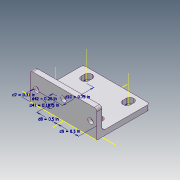
# Autodesk Inventor part: J005358
Saved by Autodesk Inventor 2015 SP1 (Build 190203100, 203)
## iProperties
Created: 2015-08-10
Material: ALUMINUM, 6061-T651
Vendor: HHMI: JRC - ID&F
Document SubType Name: Modeling
Designer: ARNOLDJ
Density: 2.7 g/cm^3
Appearance: Metal-AL-6061 (Machined)
Mass: 8.98458 g
Surface Area: 27.6253 cm^2
Volume: 3.32762 cm^3
Description: MOUNT FOR STEEL PART ON ROTARY LOCK
Project: P-201804
Part Number: J005358
RuleStatus: InUse
AfterDocSave0: file://Part Number Cleaner
LAB/DEPT: SVOBODA (LAB)
REQUESTING SCIENTIST: SOFRONIEW, NICK
SURFACE ROUGHNESS: 63 Ra
DESIGN DEPARTMENT: HHMI: JRC - ID&F
SPECIAL FINISH: NONE
ALTERED ITEM PART NUMBER: N/A
ALTERED ITEM VENDOR: N/A
ALTERED ITEM DESCRIPTION: N/A
Revision Number: -
Autodesk Inventor part; units mm, degrees
ref_plane "YZ Plane" through (0, 0, 0) normal (1, 0, 0) x (0, 1, 0)
ref_plane "XY Plane" through (0, 0, 0) normal (0, 0, 1) x (1, 0, 0)
sketch "Sketch1" plane through (0, 0, 0) normal (0, 0, 1) x (1, 0, 0)
  line L0 (20.32, -8.255) -> (-20.32, -8.255)
  line L1 (-20.32, -8.255) -> (-20.32, 8.255)
  line L2 (-20.32, 8.255) -> (20.32, 8.255)
  line L3 (20.32, 8.255) -> (20.32, -8.255)
  line L4 (20.32, -8.255) -> (-20.32, 8.255) construction
  line L5 (-20.32, -8.255) -> (20.32, 8.255) construction
  point P0 (0, 0)
  dimension "d0" = 40.64
  dimension "d1" = 16.51
  constraints: 12 end point, 2 midpoint, 2 parallel, 1 horizontal, 1 perpendicular
  measures "d0" distance of L1.end L2.end
  measures "d1" distance of L0.end L1.end
extrude "Extrusion1" add sketch "Sketch1" along normal blind 3.175
sketch "Sketch2" plane through (0, 0, 0) normal (0, 0, 1) x (1, 0, 0)
  line L0 (20.32, 8.255) -> (20.32, -8.255) projected
  line L1 (-20.32, -8.255) -> (-20.32, 8.255) projected
  line L2 (20.32, -8.255) -> (-20.32, -8.255) projected
  line L3 (20.32, -8.255) -> (-20.32, -8.255)
  line L4 (-20.32, -8.255) -> (-20.32, -5.08)
  line L5 (-20.32, -5.08) -> (20.32, -5.08)
  line L6 (20.32, -5.08) -> (20.32, -8.255)
  point P0 (0, 0)
  dimension "d4" = 3.175
  constraints: 8 end point, 2 parallel, 1 horizontal, 1 perpendicular, 1 point on line
  measures "d4" distance between parallel lines of L2 L5
extrude "Extrusion2" add sketch "Sketch2" against normal blind 29.21
sketch "Sketch3" plane through (-20.32, -8.255, 3.175) normal (0, -1, 0) x (1, 0, 0)
  line L0 (20.32, 6.477) -> (20.32, -38.862) projected
  line L1 (-8.128, -3.175) -> (48.768, -3.175) projected
  line L2 (0, 0) -> (40.64, 0) projected
  line L3 (10.0012, -11.176) -> (5.2387, -11.176)
  line L4 (5.2387, -11.176) -> (5.2387, -4.572)
  line L5 (5.2387, -4.572) -> (10.0012, -4.572)
  line L6 (10.0012, -4.572) -> (10.0012, -11.176)
  line L7 (10.0012, -11.176) -> (5.2387, -4.572) construction
  line L8 (5.2387, -11.176) -> (10.0012, -4.572) construction
  line L9 (35.4012, -11.176) -> (30.6387, -11.176)
  line L10 (30.6387, -11.176) -> (30.6387, -4.572)
  line L11 (30.6387, -4.572) -> (35.4012, -4.572)
  line L12 (35.4012, -4.572) -> (35.4012, -11.176)
  line L13 (35.4012, -11.176) -> (30.6387, -4.572) construction
  line L14 (30.6387, -11.176) -> (35.4012, -4.572) construction
  line L15 (35.4012, -30.226) -> (30.6387, -30.226)
  line L16 (30.6387, -30.226) -> (30.6387, -23.622)
  line L17 (30.6387, -23.622) -> (35.4012, -23.622)
  line L18 (35.4012, -23.622) -> (35.4012, -30.226)
  line L19 (35.4012, -30.226) -> (30.6387, -23.622) construction
  line L20 (30.6387, -30.226) -> (35.4012, -23.622) construction
  line L21 (5.2387, -30.226) -> (10.0012, -30.226)
  line L22 (10.0012, -30.226) -> (10.0012, -23.622)
  line L23 (10.0012, -23.622) -> (5.2387, -23.622)
  line L24 (5.2387, -23.622) -> (5.2387, -30.226)
  line L25 (5.2387, -30.226) -> (10.0012, -23.622) construction
  line L26 (10.0012, -30.226) -> (5.2387, -23.622) construction
  point P0 (20.32, -3.175)
  point P1 (7.62, -7.874)
  point P2 (33.02, -7.874)
  point P3 (7.62, -26.924)
  point P4 (33.02, -26.924)
  point P5 (20.32, -7.874)
  point P6 (20.32, -26.924)
  dimension "d7" = 7.874
  dimension "d8" = 12.7
  dimension "d9" = 12.7
  dimension "d10" = 19.05
  dimension "d41" = 4.7625
  dimension "d42" = 6.604
  constraints: 48 end point, 8 midpoint, 8 parallel, 6 equal length, 4 horizontal, 4 horizontal alignment, 4 perpendicular, 2 point on line, 2 vertical alignment
  measures "d7" distance from line of point (7.62, -7.874) L2
  measures "d8" distance from line of point (7.62, -7.874) L0
  measures "d9" distance from line of L0 point (33.02, -7.874)
  measures "d10" distance of point (7.62, -26.924) point (7.62, -7.874)
  measures "d41" distance of L4.end L5.end
  measures "d42" distance of L3.end L4.end
extrude "Extrusion4" cut sketch "Sketch3" against normal blind 25.4
hole "Hole1" [suppressed]
sketch "Sketch4" plane through (0, 0, 3.175) normal (0, 0, 1) x (1, 0, 0)
  point P0 (0, 0)
sketch "Sketch5" plane through (0, 0, 0) normal (0, 0, -1) x (-1, 0, 0)
  line L0 (-20.32, -8.255) -> (20.32, -8.255)
  line L1 (20.32, 7.62) -> (-20.32, 7.62)
  line L2 (0, -11.557) -> (0, 11.557) projected
  line L3 (-28.448, 0) -> (28.448, 0) projected
  line L4 (-20.32, -8.255) -> (20.32, -8.255) projected
  line L5 (20.32, -5.08) -> (20.32, 8.255) projected
  point P0 (0, 0)
  point P1 (0, 3.175)
  point P2 (-16.51, 0)
  point P3 (16.51, 0)
  dimension "d29" = 0
  dimension "d36" = 8.255
  dimension "d37" = 11.43
  dimension "d39" = 33.02
  dimension "d40" = 16.51
  constraints: 4 end point, 1 horizontal alignment
  measures "d29" distance from line of L2 point (0, 3.175)
  measures "d36" distance from line of L0 point (16.51, 0)
  measures "d37" distance from line of L0 point (0, 3.175)
  measures "d39" distance of point (16.51, 0) point (-16.51, 0)
  measures "d40" distance from line of point (16.51, 0) L2
hole "Hole2" at (0, 3.175, 0) at (16.51, 0, 0) at (-16.51, 0, 0) direction (0, 0, 1) diameter 3.2639 end through all countersink diameter 5.715 countersink angle 90
fillet "Fillet1" radius 1.5875 4 edges at (20.32, 8.255, 1.5875) (-20.32, 8.255, 1.5875) (20.32, -6.6675, -29.21) (-20.32, -6.6675, -29.21)
fillet "Fillet2" radius 1.6002 1 edges at (0, -5.08, 0)
sketch "Sketch6" plane through (-18.7325, -5.08, -29.21) normal (0, 1, 0) x (1, 0, 0)
  point P0 (18.7325, -29.21)
sketch "Sketch7" plane through (10.3187, -5.08, -8.001) normal (0, 1, 0) x (1, 0, 0)
  circle A0 centre (-23.0187, -3.302) radius 3.9688
  circle A1 centre (2.3813, -3.302) radius 3.9688
  point P0 (-23.0187, -3.302)
  point P1 (2.3813, -3.302)
  dimension "d33" = 7.9375
  constraints: 4 coincident, 2 centre point, 1 equal radius
  measures "d33" diameter of A0
extrude "Extrusion3" cut sketch "Sketch7" along normal up to surface (13.335 mm away)
fillet "Fillet3" radius 2.3622 16 edges at (-15.0813, -6.6675, -27.051) (-15.0813, -6.6675, -20.447) (-10.3188, -6.6675, -27.051) (-10.3188, -6.6675, -20.447) (15.0812, -6.6675, -27.051) (15.0812, -6.6675, -20.447) (10.3187, -6.6675, -20.447) (10.3187, -6.6675, -27.051) (15.0812, -6.661, -1.397) (15.0812, -6.6675, -8.001) (10.3187, -6.6675, -8.001) (10.3187, -6.661, -1.397) (-15.0813, -6.661, -1.397) (-10.3188, -6.661, -1.397) (-10.3188, -6.6675, -8.001) (-15.0813, -6.6675, -8.001)
body "Solid1"
